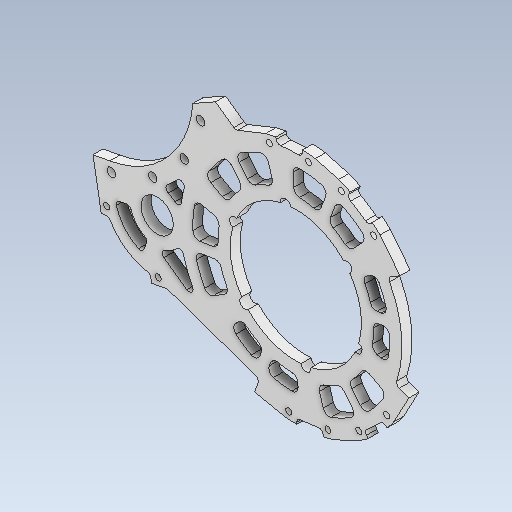
# Autodesk Inventor part: motor_h_2
Saved by Autodesk Inventor 2020 (Build 240168000, 168)
## iProperties
Created: 2020-07-14
Part Number: motor_h_2
Material: ABS Plastic
Document SubType Name: Modeling
Designer: psrobotics
Density: 1.06 g/cm^3
Appearance: Smooth - White
Author: psrobotics
Autodesk Inventor part; units mm, degrees
(part 1 of 2)
ref_plane "YZ Plane" through (0, 0, 0) normal (1, 0, 0) x (0, 1, 0)
ref_plane "XZ Plane" through (0, 0, 0) normal (0, 1, 0) x (-1, 0, 0)
ref_plane "XY Plane" through (0, 0, 0) normal (0, 0, 1) x (1, 0, 0)
sketch "Sketch1" plane through (0, 0, 0) normal (0, 0, 1) x (1, 0, 0)
  circle A0 centre (12.2297, 10.2049) radius 2.05 projected
  circle A1 centre (28.1949, -0.8291) radius 2.05 projected
  circle A2 centre (-4.0964, 14.5795) radius 2.05 projected
  circle A3 centre (-23.4396, 13.0063) radius 2.05 projected
  line L0 (35.1261, -15.125) -> (41.2511, -11.5887) projected
  line L1 (31.3473, 0.9908) -> (41.2511, -11.5887) projected
  arc A4 (31.3473, 0.9908) -> (27.4962, 4.4629) centre (-10.3402, -41.375) ccw projected
  line L2 (26.8782, 3.7142) -> (27.4962, 4.4629) projected
  arc A5 (24.1161, 3.4024) -> (26.8782, 3.7142) centre (25.3358, 4.9874) ccw projected
  arc A6 (24.1161, 3.4024) -> (16.8075, 8.1755) centre (-10.3402, -41.375) ccw projected
  arc A7 (15.9827, 10.8299) -> (16.8075, 8.1755) centre (17.7685, 9.9295) ccw projected
  line L3 (16.5842, 12.0228) -> (15.9827, 10.8299) projected
  arc A8 (16.5842, 12.0228) -> (10.8551, 14.5447) centre (-10.3402, -41.375) ccw projected
  line L4 (10.8551, 14.5447) -> (-0.736, 17.6505) projected
  arc A9 (-0.736, 17.6505) -> (-6.9585, 18.3311) centre (-10.3402, -41.375) ccw projected
  line L5 (-6.9585, 18.3311) -> (-7.034, 16.9972) projected
  arc A10 (-9.0756, 15.1108) -> (-7.034, 16.9972) centre (-9.0308, 17.1103) ccw projected
  arc A11 (-9.0756, 15.1108) -> (-17.7916, 14.6315) centre (-10.3402, -41.375) ccw projected
  arc A12 (-20.0277, 16.2826) -> (-17.7916, 14.6315) centre (-18.0553, 16.614) ccw projected
  line L6 (-20.0277, 16.2826) -> (-20.1886, 17.24) projected
  arc A13 (-20.1886, 17.24) -> (-25.2597, 16.1586) centre (-10.3402, -41.375) ccw projected
  line L7 (-25.2597, 16.1586) -> (-40.1265, 10.2163) projected
  line L8 (-40.1265, 10.2163) -> (-36.5902, 4.0913) projected
  arc A14 (35.1261, -15.125) -> (-36.5902, 4.0913) centre (-10.3402, -41.375) ccw projected
  circle A15 centre (5.5251, -95.3952) radius 2.05 projected
  circle A16 centre (-13.7974, -97.2048) radius 2.05 projected
  circle A17 centre (20.8436, -88.2521) radius 2.05 projected
  circle A18 centre (34.6501, -74.6133) radius 2.05 projected
  line L9 (-28.2963, -90.7089) -> (-30.7152, -97.3549) projected
  line L10 (-15.0425, -100.6253) -> (-30.7152, -97.3549) projected
  arc A19 (-15.0425, -100.6253) -> (-9.8606, -100.8097) centre (-10.3402, -41.375) ccw projected
  line L11 (-9.8684, -99.8389) -> (-9.8606, -100.8097) projected
  arc A20 (-7.953, -97.8245) -> (-9.8684, -99.8389) centre (-7.8685, -99.8228) ccw projected
  arc A21 (-7.953, -97.8245) -> (0.7138, -96.7831) centre (-10.3402, -41.375) ccw projected
  arc A22 (3.052, -98.2863) -> (0.7138, -96.7831) centre (1.1051, -98.7445) ccw projected
  line L12 (3.358, -99.5868) -> (3.052, -98.2863) projected
  arc A23 (3.358, -99.5868) -> (9.3677, -97.836) centre (-10.3402, -41.375) ccw projected
  line L13 (9.3677, -97.836) -> (20.2434, -92.7646) projected
  arc A24 (20.2434, -92.7646) -> (25.4476, -89.2862) centre (-10.3402, -41.375) ccw projected
  line L14 (25.4476, -89.2862) -> (24.6481, -88.2159) projected
  arc A25 (24.9994, -85.4585) -> (24.6481, -88.2159) centre (26.2504, -87.019) ccw projected
  arc A26 (24.9994, -85.4585) -> (31.3681, -79.4888) centre (-10.3402, -41.375) ccw projected
  arc A27 (34.1424, -79.3163) -> (31.3681, -79.4888) centre (32.8445, -80.838) ccw projected
  line L15 (34.1424, -79.3163) -> (34.8811, -79.9463) projected
  arc A28 (34.8811, -79.9463) -> (38.0707, -75.8583) centre (-10.3402, -41.375) ccw projected
  line L16 (38.0707, -75.8583) -> (45.6397, -61.75) projected
  line L17 (45.6397, -61.75) -> (38.9936, -59.3311) projected
  arc A29 (-28.2963, -90.7089) -> (38.9936, -59.3311) centre (-10.3402, -41.375) ccw projected
  circle A30 centre (-103.9086, -54.247) radius 2.1 projected
  circle A31 centre (-78.4226, -72.0925) radius 2.1 projected
  line L18 (-101.1564, -49.7) -> (-108.0501, -50.9156) projected
  line L19 (-107.6019, -53.4573) -> (-108.0501, -50.9156) projected
  line L20 (-106.6609, -58.794) -> (-107.6019, -53.4573) projected
  line L21 (-103.0049, -58.1494) -> (-106.6609, -58.794) projected
  arc A32 (-103.0049, -58.1494) -> (-96.5394, -66.3187) centre (-78.9982, -45.7929) ccw projected
  arc A33 (-96.5394, -66.3187) -> (-92.2867, -69.2965) centre (-78.9982, -45.7929) ccw projected
  arc A34 (-92.2867, -69.2965) -> (-82.3987, -72.578) centre (-78.9982, -45.7929) ccw projected
  line L22 (-82.3987, -72.578) -> (-81.7541, -76.234) projected
  line L23 (-81.7541, -76.234) -> (-76.4173, -75.2929) projected
  line L24 (-76.4173, -75.2929) -> (-73.8756, -74.8448) projected
  line L25 (-73.8756, -74.8448) -> (-75.0911, -67.9511) projected
  arc A35 (-101.1564, -49.7) -> (-75.0911, -67.9511) centre (-78.9982, -45.7929) ccw projected
  circle A36 centre (-111.1209, 15.0476) radius 45.5 projected
  arc A37 (-77.155, 49.6681) -> (-159.3589, 20.0812) centre (-111.1209, 15.0476) ccw projected
  circle A38 centre (-111.1209, 15.0476) radius 50
  circle A39 centre (-78.9982, -45.7929) radius 22.5
  circle A40 centre (-10.3402, -41.375) radius 52.5
  line L26 (-108.0501, -50.9156) -> (-110.8649, -34.9517)
  line L27 (-28.2963, -90.7089) -> (-73.8756, -74.8448)
  line L28 (-40.1265, 10.2163) -> (-62.337, 26.0083)
  line L29 (-88.8382, 29.4985) -> (-25.0902, -15.8273) projected
  point P0 (0, 0)
  dimension "d0" = 100
  dimension "d1" = 45
  dimension "d2" = 105
  constraints: 6 end point, 3 centre point, 3 coincident, 2 point on circle, 1 collinear, 1 parallel
  measures "d0" diameter of A38
  measures "d1" diameter of A39
  measures "d2" diameter of A40
extrude "Extrusion1" add sketch "Sketch1" along normal blind 5 contours A0 | A1 | A2 | A3 | A14 L8 L7 A13 L6 A12 A11 A10 L5 A9 L4 A8 L3 A7 A6 A5 L2 A4 L1 L0 | A40 A29 A39 A14 | A40 L29 A38 L28 L8 | A40 A39 A38 L29 | L17 L16 A28 L15 A27 A26 A25 L14 A24 L13 A23 L12 A22 A21 A20 L11 A19 L10 L9 A29 | A40 A39 A35 A38 | A39 A40 | L27 L25 A39 A40 | A38 A39 L18 L26 | L24 L23 L22 A34 A33 A32 L21 L20 L19 L18 A35 L25 | A15 | A16 | A17 | A18 | A30 | A31
sketch "Sketch2" plane through (0, 0, 5) normal (0, 0, 1) x (1, 0, 0)
  arc A0 (-20.0277, 16.2826) -> (-17.7916, 14.6315) centre (-18.0553, 16.614) ccw projected
  line L0 (-20.0277, 16.2826) -> (-20.1886, 17.24) projected
  arc A1 (-20.1886, 17.24) -> (-25.2597, 16.1586) centre (-10.3402, -41.375) ccw projected
  line L1 (-25.2597, 16.1586) -> (-40.1265, 10.2163) projected
  line L2 (-40.1265, 10.2163) -> (-62.337, 26.0083) projected
  arc A2 (-110.8649, -34.9517) -> (-62.337, 26.0083) centre (-111.1209, 15.0476) ccw projected
  line L3 (-110.8649, -34.9517) -> (-106.6609, -58.794) projected
  line L4 (-106.6609, -58.794) -> (-103.0049, -58.1494) projected
  arc A3 (-103.0049, -58.1494) -> (-82.3987, -72.578) centre (-78.9982, -45.7929) ccw projected
  line L5 (-82.3987, -72.578) -> (-81.7541, -76.234) projected
  line L6 (-81.7541, -76.234) -> (-73.8756, -74.8448) projected
  line L7 (-73.8756, -74.8448) -> (-28.2963, -90.7089) projected
  line L8 (-28.2963, -90.7089) -> (-30.7152, -97.3549) projected
  line L9 (-30.7152, -97.3549) -> (-15.0425, -100.6253) projected
  arc A4 (-15.0425, -100.6253) -> (-9.8606, -100.8097) centre (-10.3402, -41.375) ccw projected
  line L10 (-9.8606, -100.8097) -> (-9.8684, -99.8389) projected
  arc A5 (-7.953, -97.8245) -> (-9.8684, -99.8389) centre (-7.8685, -99.8228) ccw projected
  arc A6 (-7.953, -97.8245) -> (0.7138, -96.7831) centre (-10.3402, -41.375) ccw projected
  arc A7 (3.052, -98.2863) -> (0.7138, -96.7831) centre (1.1051, -98.7445) ccw projected
  line L11 (3.052, -98.2863) -> (3.358, -99.5868) projected
  arc A8 (3.358, -99.5868) -> (9.3677, -97.836) centre (-10.3402, -41.375) ccw projected
  line L12 (9.3677, -97.836) -> (20.2434, -92.7646) projected
  arc A9 (20.2434, -92.7646) -> (25.4476, -89.2862) centre (-10.3402, -41.375) ccw projected
  line L13 (25.4476, -89.2862) -> (24.6481, -88.2159) projected
  arc A10 (24.9994, -85.4585) -> (24.6481, -88.2159) centre (26.2504, -87.019) ccw projected
  arc A11 (24.9994, -85.4585) -> (31.3681, -79.4888) centre (-10.3402, -41.375) ccw projected
  arc A12 (34.1424, -79.3163) -> (31.3681, -79.4888) centre (32.8445, -80.838) ccw projected
  line L14 (34.1424, -79.3163) -> (34.8811, -79.9463) projected
  arc A13 (34.8811, -79.9463) -> (38.0707, -75.8583) centre (-10.3402, -41.375) ccw projected
  line L15 (38.0707, -75.8583) -> (45.6397, -61.75) projected
  line L16 (45.6397, -61.75) -> (38.9936, -59.3311) projected
  arc A14 (38.9936, -59.3311) -> (35.1261, -15.125) centre (-10.3402, -41.375) ccw projected
  line L17 (35.1261, -15.125) -> (41.2511, -11.5887) projected
  line L18 (41.2511, -11.5887) -> (31.3473, 0.9908) projected
  arc A15 (31.3473, 0.9908) -> (27.4962, 4.4629) centre (-10.3402, -41.375) ccw projected
  line L19 (27.4962, 4.4629) -> (26.8782, 3.7142) projected
  arc A16 (24.1161, 3.4024) -> (26.8782, 3.7142) centre (25.3358, 4.9874) ccw projected
  arc A17 (24.1161, 3.4024) -> (16.8075, 8.1755) centre (-10.3402, -41.375) ccw projected
  arc A18 (15.9827, 10.8299) -> (16.8075, 8.1755) centre (17.7685, 9.9295) ccw projected
  line L20 (15.9827, 10.8299) -> (16.5842, 12.0228) projected
  arc A19 (16.5842, 12.0228) -> (10.8551, 14.5447) centre (-10.3402, -41.375) ccw projected
  line L21 (10.8551, 14.5447) -> (-0.736, 17.6505) projected
  arc A20 (-0.736, 17.6505) -> (-6.9585, 18.3311) centre (-10.3402, -41.375) ccw projected
  line L22 (-6.9585, 18.3311) -> (-7.034, 16.9972) projected
  arc A21 (-9.0756, 15.1108) -> (-7.034, 16.9972) centre (-9.0308, 17.1103) ccw projected
  arc A22 (-9.0756, 15.1108) -> (-17.7916, 14.6315) centre (-10.3402, -41.375) ccw projected
  line L23 (-111.1209, 15.0476) -> (-102.4384, -34.1927)
  line L24 (-102.4384, -34.1927) -> (-110.7406, -35.6566)
  line L25 (-110.8649, -34.9517) -> (-106.6609, -58.794) projected
  point P0 (0, 0)
  constraints: 4 end point, 2 perpendicular, 1 point on circle, 1 point on line
extrude "Extrusion2" cut sketch "Sketch2" against normal blind 5 contours L24 L3 A2
sketch "Sketch3" plane through (0, 0, 5) normal (0, 0, 1) x (1, 0, 0)
  circle A0 centre (-23.4396, 13.0063) radius 2.05 projected
  circle A1 centre (-4.0964, 14.5795) radius 2.05 projected
  circle A2 centre (12.2297, 10.2049) radius 2.05 projected
  circle A3 centre (28.1949, -0.8291) radius 2.05 projected
  circle A4 centre (34.6501, -74.6133) radius 2.05 projected
  circle A5 centre (20.8436, -88.2521) radius 2.05 projected
  circle A6 centre (5.5251, -95.3952) radius 2.05 projected
  circle A7 centre (-13.7974, -97.2048) radius 2.05 projected
  circle A8 centre (-78.4226, -72.0925) radius 2.1 projected
  circle A9 centre (-103.9086, -54.247) radius 2.1 projected
  point P0 (0, 0)
hole "Hole1" at (-23.4396, 13.0063, 5) at (-4.0964, 14.5795, 5) at (12.2297, 10.2049, 5) at (28.1949, -0.8291, 5) at (34.6501, -74.6133, 5) at (20.8436, -88.2521, 5) at (5.5251, -95.3952, 5) at (-13.7974, -97.2048, 5) at (-78.4226, -72.0925, 5) at (-103.9086, -54.247, 5) direction (0, 0, -1) diameter 3 depth 17
sketch "Sketch6" plane through (0, 0, 5) normal (0, 0, 1) x (1, 0, 0)
  circle A0 centre (-10.3402, -41.375) radius 4.075 projected
  circle A1 centre (-10.3402, -41.375) radius 32.5 projected
  circle A2 centre (-10.3402, -41.375) radius 32.5
  point P0 (0, 0)
  dimension "d16" = 65
  constraints: 1 centre point, 1 coincident
  measures "d16" diameter of A2
extrude "Extrusion4" cut sketch "Sketch6" against normal blind 5 contours A0 | A1
chamfer "Chamfer1" distance 15 angle 45 1 edges at (-62.337, 26.0083, 2.5)
sketch "Sketch7" plane through (0, 0, 5) normal (0, 0, 1) x (1, 0, 0)
  circle A0 centre (-78.9982, -45.7929) radius 4.075 projected
  circle A1 centre (-78.9982, -45.7929) radius 8
  point P0 (0, 0)
  dimension "d22" = 16
  constraints: 1 centre point, 1 coincident
  measures "d22" diameter of A1
extrude "Extrusion5" cut sketch "Sketch7" against normal blind 5 contours A0 | A1
sketch "Sketch8" plane through (0, 0, 5) normal (0, 0, 1) x (1, 0, 0)
  circle A0 centre (-78.9982, -45.7929) radius 8 projected
  line L0 (-61.2813, 11.0455) -> (-50.1121, 17.3163) projected
  arc A1 (-102.4384, -34.1927) -> (-61.2813, 11.0455) centre (-111.1209, 15.0476) ccw projected
  line L1 (-102.4384, -34.1927) -> (-110.7406, -35.6566) projected
  line L2 (-110.7406, -35.6566) -> (-106.6609, -58.794) projected
  line L3 (-106.6609, -58.794) -> (-103.0049, -58.1494) projected
  arc A2 (-103.0049, -58.1494) -> (-82.3987, -72.578) centre (-78.9982, -45.7929) ccw projected
  line L4 (-82.3987, -72.578) -> (-81.7541, -76.234) projected
  line L5 (-81.7541, -76.234) -> (-73.8756, -74.8448) projected
  line L6 (-73.8756, -74.8448) -> (-28.2963, -90.7089) projected
  line L7 (-28.2963, -90.7089) -> (-30.7152, -97.3549) projected
  line L8 (-30.7152, -97.3549) -> (-15.0425, -100.6253) projected
  arc A3 (-15.0425, -100.6253) -> (-9.8606, -100.8097) centre (-10.3402, -41.375) ccw projected
  line L9 (-9.8606, -100.8097) -> (-9.8684, -99.8389) projected
  arc A4 (-7.953, -97.8245) -> (-9.8684, -99.8389) centre (-7.8685, -99.8228) ccw projected
  arc A5 (-7.953, -97.8245) -> (0.7138, -96.7831) centre (-10.3402, -41.375) ccw projected
  arc A6 (3.052, -98.2863) -> (0.7138, -96.7831) centre (1.1051, -98.7445) ccw projected
  line L10 (3.052, -98.2863) -> (3.358, -99.5868) projected
  arc A7 (3.358, -99.5868) -> (9.3677, -97.836) centre (-10.3402, -41.375) ccw projected
  line L11 (9.3677, -97.836) -> (20.2434, -92.7646) projected
  arc A8 (20.2434, -92.7646) -> (25.4476, -89.2862) centre (-10.3402, -41.375) ccw projected
  line L12 (25.4476, -89.2862) -> (24.6481, -88.2159) projected
  arc A9 (24.9994, -85.4585) -> (24.6481, -88.2159) centre (26.2504, -87.019) ccw projected
  arc A10 (24.9994, -85.4585) -> (31.3681, -79.4888) centre (-10.3402, -41.375) ccw projected
  arc A11 (34.1424, -79.3163) -> (31.3681, -79.4888) centre (32.8445, -80.838) ccw projected
  line L13 (34.1424, -79.3163) -> (34.8811, -79.9463) projected
  arc A12 (34.8811, -79.9463) -> (38.0707, -75.8583) centre (-10.3402, -41.375) ccw projected
  line L14 (38.0707, -75.8583) -> (45.6397, -61.75) projected
  line L15 (45.6397, -61.75) -> (38.9936, -59.3311) projected
  arc A13 (38.9936, -59.3311) -> (35.1261, -15.125) centre (-10.3402, -41.375) ccw projected
  line L16 (35.1261, -15.125) -> (41.2511, -11.5887) projected
  line L17 (41.2511, -11.5887) -> (31.3473, 0.9908) projected
  arc A14 (31.3473, 0.9908) -> (27.4962, 4.4629) centre (-10.3402, -41.375) ccw projected
  line L18 (27.4962, 4.4629) -> (26.8782, 3.7142) projected
  arc A15 (24.1161, 3.4024) -> (26.8782, 3.7142) centre (25.3358, 4.9874) ccw projected
  arc A16 (24.1161, 3.4024) -> (16.8075, 8.1755) centre (-10.3402, -41.375) ccw projected
  arc A17 (15.9827, 10.8299) -> (16.8075, 8.1755) centre (17.7685, 9.9295) ccw projected
  line L19 (15.9827, 10.8299) -> (16.5842, 12.0228) projected
  arc A18 (16.5842, 12.0228) -> (10.8551, 14.5447) centre (-10.3402, -41.375) ccw projected
  line L20 (10.8551, 14.5447) -> (-0.736, 17.6505) projected
  arc A19 (-0.736, 17.6505) -> (-6.9585, 18.3311) centre (-10.3402, -41.375) ccw projected
  line L21 (-6.9585, 18.3311) -> (-7.034, 16.9972) projected
  arc A20 (-9.0756, 15.1108) -> (-7.034, 16.9972) centre (-9.0308, 17.1103) ccw projected
  arc A21 (-9.0756, 15.1108) -> (-17.7916, 14.6315) centre (-10.3402, -41.375) ccw projected
  arc A22 (-20.0277, 16.2826) -> (-17.7916, 14.6315) centre (-18.0553, 16.614) ccw projected
  line L22 (-20.0277, 16.2826) -> (-20.1886, 17.24) projected
  arc A23 (-20.1886, 17.24) -> (-25.2597, 16.1586) centre (-10.3402, -41.375) ccw projected
  line L23 (-25.2597, 16.1586) -> (-40.1265, 10.2163) projected
  line L24 (-40.1265, 10.2163) -> (-50.1121, 17.3163) projected
  circle A24 centre (-103.9086, -54.247) radius 1.5 projected
  circle A25 centre (-13.7974, -97.2048) radius 1.5 projected
  circle A26 centre (20.8436, -88.2521) radius 1.5 projected
  circle A27 centre (28.1949, -0.8291) radius 1.5 projected
  circle A28 centre (-4.0964, 14.5795) radius 1.5 projected
  circle A29 centre (-23.4396, 13.0063) radius 1.5 projected
  circle A30 centre (12.2297, 10.2049) radius 1.5 projected
  circle A31 centre (34.6501, -74.6133) radius 1.5 projected
  circle A32 centre (5.5251, -95.3952) radius 1.5 projected
  circle A33 centre (-78.4226, -72.0925) radius 1.5 projected
  circle A34 centre (-10.3402, -41.375) radius 32.5 projected
  circle A35 centre (-111.1209, 15.0476) radius 50
  circle A36 centre (-111.1209, 15.0476) radius 59
  line L25 (-110.7406, -35.6566) -> (-102.4384, -34.1927) projected
  line L26 (-111.1209, 15.0476) -> (-102.4384, -34.1927)
  line L27 (-102.4384, -34.1927) -> (-100.8756, -43.056)
  circle A37 centre (-101.657, -38.6244) radius 2.1
  circle A38 centre (-81.1726, -30.4864) radius 2.1
  circle A39 centre (-65.5868, -14.9006) radius 2.1
  circle A40 centre (-57.4488, 5.5838) radius 2.1
  point P0 (0, 0)
  dimension "d26" = 118
  dimension "d25" = 100
  dimension "d27" = 4.2
  dimension "d30" = 70
  constraints: 5 centre point, 4 end point, 2 coincident, 1 midpoint, 1 perpendicular, 1 point on line, 10 other
  measures "d25" diameter of A35
  measures "d27" diameter of A37
extrude "Extrusion6" cut sketch "Sketch8" against normal blind 5 contours A37 L27 | L27 A37 | A38 | A39 | A40
sketch "Sketch10" plane through (0, 0, 5) normal (0, 0, 1) x (1, 0, 0)
  circle A0 centre (-10.3402, -41.375) radius 32.5 projected
  circle A1 centre (-81.1726, -30.4864) radius 2.1 projected
  circle A2 centre (-65.5868, -14.9006) radius 2.1 projected
  circle A3 centre (-101.657, -38.6244) radius 2.1 projected
  circle A4 centre (-57.4488, 5.5838) radius 2.1 projected
  circle A5 centre (-78.9982, -45.7929) radius 8 projected
  line L0 (-61.2813, 11.0455) -> (-50.1121, 17.3163) projected
  arc A6 (-102.4384, -34.1927) -> (-61.2813, 11.0455) centre (-111.1209, 15.0476) ccw projected
  line L1 (-102.4384, -34.1927) -> (-110.7406, -35.6566) projected
  line L2 (-110.7406, -35.6566) -> (-106.6609, -58.794) projected
  line L3 (-106.6609, -58.794) -> (-103.0049, -58.1494) projected
  arc A7 (-103.0049, -58.1494) -> (-82.3987, -72.578) centre (-78.9982, -45.7929) ccw projected
  line L4 (-82.3987, -72.578) -> (-81.7541, -76.234) projected
  line L5 (-81.7541, -76.234) -> (-73.8756, -74.8448) projected
  line L6 (-73.8756, -74.8448) -> (-28.2963, -90.7089) projected
  line L7 (-28.2963, -90.7089) -> (-30.7152, -97.3549) projected
  line L8 (-30.7152, -97.3549) -> (-15.0425, -100.6253) projected
  arc A8 (-15.0425, -100.6253) -> (-9.8606, -100.8097) centre (-10.3402, -41.375) ccw projected
  line L9 (-9.8606, -100.8097) -> (-9.8684, -99.8389) projected
  arc A9 (-7.953, -97.8245) -> (-9.8684, -99.8389) centre (-7.8685, -99.8228) ccw projected
  arc A10 (-7.953, -97.8245) -> (0.7138, -96.7831) centre (-10.3402, -41.375) ccw projected
  arc A11 (3.052, -98.2863) -> (0.7138, -96.7831) centre (1.1051, -98.7445) ccw projected
  line L10 (3.052, -98.2863) -> (3.358, -99.5868) projected
  arc A12 (3.358, -99.5868) -> (9.3677, -97.836) centre (-10.3402, -41.375) ccw projected
  line L11 (9.3677, -97.836) -> (20.2434, -92.7646) projected
  arc A13 (20.2434, -92.7646) -> (25.4476, -89.2862) centre (-10.3402, -41.375) ccw projected
  line L12 (25.4476, -89.2862) -> (24.6481, -88.2159) projected
  arc A14 (24.9994, -85.4585) -> (24.6481, -88.2159) centre (26.2504, -87.019) ccw projected
  arc A15 (24.9994, -85.4585) -> (31.3681, -79.4888) centre (-10.3402, -41.375) ccw projected
  arc A16 (34.1424, -79.3163) -> (31.3681, -79.4888) centre (32.8445, -80.838) ccw projected
  line L13 (34.1424, -79.3163) -> (34.8811, -79.9463) projected
  arc A17 (34.8811, -79.9463) -> (38.0707, -75.8583) centre (-10.3402, -41.375) ccw projected
  line L14 (38.0707, -75.8583) -> (45.6397, -61.75) projected
  line L15 (45.6397, -61.75) -> (38.9936, -59.3311) projected
  arc A18 (38.9936, -59.3311) -> (35.1261, -15.125) centre (-10.3402, -41.375) ccw projected
  line L16 (35.1261, -15.125) -> (41.2511, -11.5887) projected
  line L17 (41.2511, -11.5887) -> (31.3473, 0.9908) projected
  arc A19 (31.3473, 0.9908) -> (27.4962, 4.4629) centre (-10.3402, -41.375) ccw projected
  line L18 (27.4962, 4.4629) -> (26.8782, 3.7142) projected
  arc A20 (24.1161, 3.4024) -> (26.8782, 3.7142) centre (25.3358, 4.9874) ccw projected
  arc A21 (24.1161, 3.4024) -> (16.8075, 8.1755) centre (-10.3402, -41.375) ccw projected
  arc A22 (15.9827, 10.8299) -> (16.8075, 8.1755) centre (17.7685, 9.9295) ccw projected
  line L19 (15.9827, 10.8299) -> (16.5842, 12.0228) projected
  arc A23 (16.5842, 12.0228) -> (10.8551, 14.5447) centre (-10.3402, -41.375) ccw projected
  line L20 (10.8551, 14.5447) -> (-0.736, 17.6505) projected
  arc A24 (-0.736, 17.6505) -> (-6.9585, 18.3311) centre (-10.3402, -41.375) ccw projected
  line L21 (-6.9585, 18.3311) -> (-7.034, 16.9972) projected
  arc A25 (-9.0756, 15.1108) -> (-7.034, 16.9972) centre (-9.0308, 17.1103) ccw projected
  arc A26 (-9.0756, 15.1108) -> (-17.7916, 14.6315) centre (-10.3402, -41.375) ccw projected
  arc A27 (-20.0277, 16.2826) -> (-17.7916, 14.6315) centre (-18.0553, 16.614) ccw projected
  line L22 (-20.0277, 16.2826) -> (-20.1886, 17.24) projected
  arc A28 (-20.1886, 17.24) -> (-25.2597, 16.1586) centre (-10.3402, -41.375) ccw projected
  line L23 (-25.2597, 16.1586) -> (-40.1265, 10.2163) projected
  line L24 (-40.1265, 10.2163) -> (-50.1121, 17.3163) projected
  circle A29 centre (-103.9086, -54.247) radius 1.5 projected
  circle A30 centre (-13.7974, -97.2048) radius 1.5 projected
  circle A31 centre (20.8436, -88.2521) radius 1.5 projected
  circle A32 centre (28.1949, -0.8291) radius 1.5 projected
  circle A33 centre (-4.0964, 14.5795) radius 1.5 projected
  circle A34 centre (-23.4396, 13.0063) radius 1.5 projected
  circle A35 centre (12.2297, 10.2049) radius 1.5 projected
  circle A36 centre (34.6501, -74.6133) radius 1.5 projected
  circle A37 centre (5.5251, -95.3952) radius 1.5 projected
  circle A38 centre (-78.4226, -72.0925) radius 1.5 projected
  circle A39 centre (-10.3402, -41.375) radius 32.5 projected
  circle A40 centre (28.1949, -0.8291) radius 1.5 projected
  line L25 (-10.3402, -41.375) -> (28.1949, -0.8291)
  circle A41 centre (-10.3402, -41.375) radius 32.5
  circle A42 centre (-10.3402, -41.375) radius 38.5
  circle A43 centre (-10.3402, -41.375) radius 46.5
  circle A44 centre (-10.3402, -41.375) radius 51
  line L26 (-10.3402, -41.375) -> (39.2416, -53.3183)
  line L27 (-10.3402, -41.375) -> (33.1646, -14.7606)
  line L28 (-10.3402, -41.375) -> (-11.6366, 9.6085)
  line L29 (-10.3402, -41.375) -> (24.7939, -4.4075)
  line L30 (-10.3402, -41.375) -> (-55.1414, -17.0059)
  line L31 (-10.3402, -41.375) -> (-24.7879, 7.5358)
  line L32 (-10.3402, -41.375) -> (-53.8451, -67.9894)
  line L33 (-10.3402, -41.375) -> (-59.922, -29.4317)
  line L34 (-10.3402, -41.375) -> (-9.0439, -92.3585)
  line L35 (-10.3402, -41.375) -> (-45.4743, -78.3425)
  line L36 (-10.3402, -41.375) -> (34.461, -65.7441)
  line L37 (-10.3402, -41.375) -> (4.1075, -90.2858)
  point P0 (0, 0)
  point P1 (-11.3188, -2.8874)
  point P2 (16.1826, -13.4682)
  point P3 (24.7939, -4.4075)
  point P4 (-44.1607, -22.9787)
  point P5 (-21.2468, -4.4522)
  point P6 (-43.1821, -61.4663)
  point P7 (-47.7696, -32.359)
  point P8 (-36.863, -69.2818)
  point P9 (-42.3743, -75.0806)
  point P10 (-9.1582, -87.86)
  point P11 (-9.3616, -79.8626)
  point P12 (23.4803, -59.7713)
  point P13 (0.5664, -78.2978)
  point P14 (29.326, -17.1089)
  point P15 (22.5017, -21.2837)
  point P16 (27.0892, -50.391)
  point P17 (34.8667, -52.2645)
  dimension "d38" = 65
  dimension "d39" = 77
  dimension "d40" = 93
  dimension "d41" = 102
  dimension "d42" = 60
  dimension "d43" = 15
  dimension "d46" = 360
  constraints: 26 end point, 4 centre point, 4 coincident, 2 point on circle, 31 other
  measures "d38" diameter of A41
  measures "d39" diameter of A42
  measures "d40" diameter of A43
  measures "d41" diameter of A44
  measures "d42" angle of L25 L26
  measures "d43" angle of L25 L27
extrude "Extrusion8" cut sketch "Sketch10" against normal blind 5 contours L27 A43 L26 A42 | A42 L28 A43 L25 | L36 A43 L37 A42 | A43 L28 A44 L25 | L30 A43 L31 A42 | L32 A43 L33 A42 | L34 A43 L35 A42 | L36 A44 L37 A43 | L30 A44 L31 A43 | L32 A44 L33 A43
sketch "Sketch11" plane through (0, 0, 5) normal (0, 0, 1) x (1, 0, 0)
  line L0 (-9.3616, -79.8626) -> (-9.1582, -87.86) projected
  arc A0 (-42.3743, -75.0806) -> (-9.1582, -87.86) centre (-10.3402, -41.375) ccw projected
  line L1 (-42.3743, -75.0806) -> (-36.863, -69.2818) projected
  arc A1 (-36.863, -69.2818) -> (-9.3616, -79.8626) centre (-10.3402, -41.375) ccw projected
  arc A2 (24.7939, -4.4075) -> (-11.6366, 9.6085) centre (-10.3402, -41.375) ccw projected
  line L2 (24.7939, -4.4075) -> (16.1826, -13.4682) projected
  arc A3 (16.1826, -13.4682) -> (-11.3188, -2.8874) centre (-10.3402, -41.375) ccw projected
  line L3 (-11.3188, -2.8874) -> (-11.6366, 9.6085) projected
  line L4 (23.4803, -59.7713) -> (34.461, -65.7441) projected
  arc A4 (4.1075, -90.2858) -> (34.461, -65.7441) centre (-10.3402, -41.375) ccw projected
  line L5 (4.1075, -90.2858) -> (0.5664, -78.2978) projected
  arc A5 (0.5664, -78.2978) -> (23.4803, -59.7713) centre (-10.3402, -41.375) ccw projected
  arc A6 (-47.7696, -32.359) -> (-43.1821, -61.4663) centre (-10.3402, -41.375) ccw projected
  line L6 (-43.1821, -61.4663) -> (-53.8451, -67.9894) projected
  arc A7 (-59.922, -29.4317) -> (-53.8451, -67.9894) centre (-10.3402, -41.375) ccw projected
  line L7 (-59.922, -29.4317) -> (-47.7696, -32.359) projected
  arc A8 (-21.2468, -4.4522) -> (-44.1607, -22.9787) centre (-10.3402, -41.375) ccw projected
  line L8 (-44.1607, -22.9787) -> (-55.1414, -17.0059) projected
  arc A9 (-24.7879, 7.5358) -> (-55.1414, -17.0059) centre (-10.3402, -41.375) ccw projected
  line L9 (-24.7879, 7.5358) -> (-21.2468, -4.4522) projected
  arc A10 (34.8667, -52.2645) -> (29.326, -17.1089) centre (-10.3402, -41.375) ccw projected
  line L10 (34.8667, -52.2645) -> (27.0892, -50.391) projected
  arc A11 (27.0892, -50.391) -> (22.5017, -21.2837) centre (-10.3402, -41.375) ccw projected
  line L11 (22.5017, -21.2837) -> (29.326, -17.1089) projected
  circle A12 centre (-81.1726, -30.4864) radius 2.1 projected
  circle A13 centre (-65.5868, -14.9006) radius 2.1 projected
  circle A14 centre (-101.657, -38.6244) radius 2.1 projected
  circle A15 centre (-57.4488, 5.5838) radius 2.1 projected
  circle A16 centre (-78.9982, -45.7929) radius 8 projected
  line L12 (-61.2813, 11.0455) -> (-50.1121, 17.3163) projected
  arc A17 (-102.4384, -34.1927) -> (-61.2813, 11.0455) centre (-111.1209, 15.0476) ccw projected
  line L13 (-102.4384, -34.1927) -> (-110.7406, -35.6566) projected
  line L14 (-110.7406, -35.6566) -> (-106.6609, -58.794) projected
  line L15 (-106.6609, -58.794) -> (-103.0049, -58.1494) projected
  arc A18 (-103.0049, -58.1494) -> (-82.3987, -72.578) centre (-78.9982, -45.7929) ccw projected
  line L16 (-82.3987, -72.578) -> (-81.7541, -76.234) projected
  line L17 (-81.7541, -76.234) -> (-73.8756, -74.8448) projected
  line L18 (-73.8756, -74.8448) -> (-28.2963, -90.7089) projected
  line L19 (-28.2963, -90.7089) -> (-30.7152, -97.3549) projected
  line L20 (-30.7152, -97.3549) -> (-15.0425, -100.6253) projected
  arc A19 (-15.0425, -100.6253) -> (-9.8606, -100.8097) centre (-10.3402, -41.375) ccw projected
  line L21 (-9.8606, -100.8097) -> (-9.8684, -99.8389) projected
  arc A20 (-7.953, -97.8245) -> (-9.8684, -99.8389) centre (-7.8685, -99.8228) ccw projected
  arc A21 (-7.953, -97.8245) -> (0.7138, -96.7831) centre (-10.3402, -41.375) ccw projected
  arc A22 (3.052, -98.2863) -> (0.7138, -96.7831) centre (1.1051, -98.7445) ccw projected
  line L22 (3.052, -98.2863) -> (3.358, -99.5868) projected
  arc A23 (3.358, -99.5868) -> (9.3677, -97.836) centre (-10.3402, -41.375) ccw projected
  line L23 (9.3677, -97.836) -> (20.2434, -92.7646) projected
  arc A24 (20.2434, -92.7646) -> (25.4476, -89.2862) centre (-10.3402, -41.375) ccw projected
  line L24 (25.4476, -89.2862) -> (24.6481, -88.2159) projected
  arc A25 (24.9994, -85.4585) -> (24.6481, -88.2159) centre (26.2504, -87.019) ccw projected
  arc A26 (24.9994, -85.4585) -> (31.3681, -79.4888) centre (-10.3402, -41.375) ccw projected
  arc A27 (34.1424, -79.3163) -> (31.3681, -79.4888) centre (32.8445, -80.838) ccw projected
  line L25 (34.1424, -79.3163) -> (34.8811, -79.9463) projected
  arc A28 (34.8811, -79.9463) -> (38.0707, -75.8583) centre (-10.3402, -41.375) ccw projected
  line L26 (38.0707, -75.8583) -> (45.6397, -61.75) projected
  line L27 (45.6397, -61.75) -> (38.9936, -59.3311) projected
  arc A29 (38.9936, -59.3311) -> (35.1261, -15.125) centre (-10.3402, -41.375) ccw projected
  line L28 (35.1261, -15.125) -> (41.2511, -11.5887) projected
  line L29 (41.2511, -11.5887) -> (31.3473, 0.9908) projected
  arc A30 (31.3473, 0.9908) -> (27.4962, 4.4629) centre (-10.3402, -41.375) ccw projected
  line L30 (27.4962, 4.4629) -> (26.8782, 3.7142) projected
  arc A31 (24.1161, 3.4024) -> (26.8782, 3.7142) centre (25.3358, 4.9874) ccw projected
  arc A32 (24.1161, 3.4024) -> (16.8075, 8.1755) centre (-10.3402, -41.375) ccw projected
  arc A33 (15.9827, 10.8299) -> (16.8075, 8.1755) centre (17.7685, 9.9295) ccw projected
  line L31 (15.9827, 10.8299) -> (16.5842, 12.0228) projected
  arc A34 (16.5842, 12.0228) -> (10.8551, 14.5447) centre (-10.3402, -41.375) ccw projected
  line L32 (10.8551, 14.5447) -> (-0.736, 17.6505) projected
  arc A35 (-0.736, 17.6505) -> (-6.9585, 18.3311) centre (-10.3402, -41.375) ccw projected
  line L33 (-6.9585, 18.3311) -> (-7.034, 16.9972) projected
  arc A36 (-9.0756, 15.1108) -> (-7.034, 16.9972) centre (-9.0308, 17.1103) ccw projected
  arc A37 (-9.0756, 15.1108) -> (-17.7916, 14.6315) centre (-10.3402, -41.375) ccw projected
  arc A38 (-20.0277, 16.2826) -> (-17.7916, 14.6315) centre (-18.0553, 16.614) ccw projected
  line L34 (-20.0277, 16.2826) -> (-20.1886, 17.24) projected
  arc A39 (-20.1886, 17.24) -> (-25.2597, 16.1586) centre (-10.3402, -41.375) ccw projected
  line L35 (-25.2597, 16.1586) -> (-40.1265, 10.2163) projected
  line L36 (-40.1265, 10.2163) -> (-50.1121, 17.3163) projected
  circle A40 centre (-103.9086, -54.247) radius 1.5 projected
  circle A41 centre (-13.7974, -97.2048) radius 1.5 projected
  circle A42 centre (20.8436, -88.2521) radius 1.5 projected
  circle A43 centre (28.1949, -0.8291) radius 1.5 projected
  circle A44 centre (-4.0964, 14.5795) radius 1.5 projected
  circle A45 centre (-23.4396, 13.0063) radius 1.5 projected
  circle A46 centre (12.2297, 10.2049) radius 1.5 projected
  circle A47 centre (34.6501, -74.6133) radius 1.5 projected
  circle A48 centre (5.5251, -95.3952) radius 1.5 projected
  circle A49 centre (-78.4226, -72.0925) radius 1.5 projected
  circle A50 centre (-10.3402, -41.375) radius 32.5 projected
  line L37 (-10.3402, -41.375) -> (27.6903, -35.3811)
  line L38 (27.6903, -35.3811) -> (35.5928, -34.1356)
  arc A51 (34.8667, -52.2645) -> (29.326, -17.1089) centre (-10.3402, -41.375) ccw projected
  line L39 (35.5928, -34.1356) -> (27.6903, -35.3811) construction
  line L40 (35.2036, -31.6661) -> (27.3011, -32.9116)
  line L41 (28.0796, -37.8506) -> (35.982, -36.6051)
  arc A52 (35.982, -36.6051) -> (35.2036, -31.6661) centre (35.5928, -34.1356) ccw
  arc A53 (27.3011, -32.9116) -> (28.0796, -37.8506) centre (27.6903, -35.3811) ccw
  arc A54 (0.5664, -78.2978) -> (23.4803, -59.7713) centre (-10.3402, -41.375) ccw projected
  line L42 (13.8659, -71.3135) -> (21.7251, -81.0338)
  arc A55 (4.1075, -90.2858) -> (34.461, -65.7441) centre (-10.3402, -41.375) ccw projected
  line L43 (13.8659, -71.3135) -> (21.7251, -81.0338) construction
  line L44 (11.9219, -72.8853) -> (19.781, -82.6056)
  line L45 (23.6691, -79.4619) -> (15.81, -69.7417)
  arc A56 (15.81, -69.7417) -> (11.9219, -72.8853) centre (13.8659, -71.3135) ccw
  arc A57 (19.781, -82.6056) -> (23.6691, -79.4619) centre (21.7251, -81.0338) ccw
  line L46 (3.4842, -5.4426) -> (7.9727, 6.2237) construction
  line L47 (5.8175, -6.3403) -> (10.3059, 5.326)
  line L48 (5.6394, 7.1214) -> (1.1509, -4.5449)
  arc A58 (1.1509, -4.5449) -> (5.8175, -6.3403) centre (3.4842, -5.4426) ccw
  arc A59 (10.3059, 5.326) -> (5.6394, 7.1214) centre (7.9727, 6.2237) ccw
  line L49 (-34.5464, -11.4365) -> (-42.4055, -1.7162) construction
  arc A60 (-24.7879, 7.5358) -> (-55.1414, -17.0059) centre (-10.3402, -41.375) ccw projected
  line L50 (-32.6023, -9.8647) -> (-40.4614, -0.1444)
  line L51 (-44.3495, -3.2881) -> (-36.4904, -13.0083)
  arc A61 (-36.4904, -13.0083) -> (-32.6023, -9.8647) centre (-34.5464, -11.4365) ccw
  arc A62 (-40.4614, -0.1444) -> (-44.3495, -3.2881) centre (-42.4055, -1.7162) ccw
  arc A63 (-47.7696, -32.359) -> (-43.1821, -61.4663) centre (-10.3402, -41.375) ccw projected
  line L52 (-48.3708, -47.3689) -> (-60.7184, -49.315) construction
  arc A64 (-59.922, -29.4317) -> (-53.8451, -67.9894) centre (-10.3402, -41.375) ccw projected
  line L53 (-48.76, -44.8994) -> (-61.1076, -46.8454)
  line L54 (-60.3291, -51.7845) -> (-47.9816, -49.8384)
  arc A65 (-47.9816, -49.8384) -> (-48.76, -44.8994) centre (-48.3708, -47.3689) ccw
  arc A66 (-61.1076, -46.8454) -> (-60.3291, -51.7845) centre (-60.7184, -49.315) ccw
  arc A67 (-36.863, -69.2818) -> (-9.3616, -79.8626) centre (-10.3402, -41.375) ccw projected
  line L55 (-24.1646, -77.3074) -> (-27.0372, -84.7738) construction
  line L56 (-26.4979, -76.4097) -> (-29.3705, -83.8761)
  line L57 (-24.704, -85.6715) -> (-21.8314, -78.2051)
  arc A68 (-21.8314, -78.2051) -> (-26.4979, -76.4097) centre (-24.1646, -77.3074) ccw
  arc A69 (-29.3705, -83.8761) -> (-24.704, -85.6715) centre (-27.0372, -84.7738) ccw
  point P0 (0, 0)
  point P1 (31.6416, -34.7584)
  point P2 (17.7955, -76.1736)
  point P3 (5.7284, 0.3905)
  point P4 (-38.4759, -6.5764)
  point P5 (-54.5446, -48.3419)
  point P6 (-25.6009, -81.0406)
  point P7 (5.7871, -6.4156)
  point P8 (10.2839, 5.2688)
  point P9 (5.6174, 7.0642)
  point P10 (1.123, -4.6212)
  point P11 (-32.5523, -9.9286)
  point P12 (-40.4229, -0.1921)
  point P13 (-44.311, -3.3357)
  point P14 (-36.4384, -13.0706)
  point P15 (-48.6796, -44.888)
  point P16 (-61.047, -46.8359)
  point P17 (-60.2686, -51.7749)
  point P18 (-47.9016, -49.8245)
  point P19 (-26.4675, -76.3344)
  point P20 (-29.3464, -83.8134)
  point P21 (-24.6798, -85.6088)
  point P22 (-21.8035, -78.1288)
  point P23 (15.7579, -69.6794)
  point P24 (11.8719, -72.8214)
  point P25 (19.7424, -82.5579)
  point P26 (23.6306, -79.4143)
  point P27 (27.9992, -37.862)
  point P28 (35.9156, -36.6156)
  point P29 (35.1371, -31.6766)
  point P30 (27.2212, -32.9255)
  dimension "d50" = 5
  dimension "d51" = 5
  dimension "d52" = 5
  dimension "d53" = 5
  dimension "d54" = 5
  dimension "d55" = 5
  constraints: 54 end point, 43 point on circle, 24 tangent, 12 centre point, 6 midpoint, 6 parallel
  measures "d50" diameter of A53
  measures "d51" diameter of A57
  measures "d52" diameter of A59
  measures "d53" diameter of A62
  measures "d54" diameter of A66
  measures "d55" diameter of A69
extrude "Extrusion9" add sketch "Sketch11" against normal blind 5 contours A68 L57 A0 L56 A1 | L47 A58 A3 L48 A2 | A56 L45 A4 L42 A5 | L42 A4 L44 A56 A5 | A6 A65 L54 A7 L53 | A8 A61 L51 A9 L50 | L41 A53 A11 L38 A10 | L38 A11 A53 L40 A10
sketch "Sketch12" plane through (0, 0, 5) normal (0, 0, 1) x (1, 0, 0)
  line L0 (-133.6423, 43.9922) -> (-138.6873, 49.6358) projected
  arc A0 (-138.1583, 54.1018) -> (-138.6873, 49.6358) centre (-136.4507, 51.6352) ccw projected
  arc A1 (-131.6901, 57.863) -> (-138.1583, 54.1018) centre (-111.1209, 15.0476) ccw projected
  arc A2 (-127.6054, 56.2727) -> (-131.6901, 57.863) centre (-130.391, 55.1589) ccw projected
  line L1 (-127.6054, 56.2727) -> (-124.8131, 49.2897) projected
  arc A3 (-126.2627, 45.4898) -> (-124.8131, 49.2897) centre (-127.5987, 48.1759) ccw projected
  arc A4 (-126.2627, 45.4898) -> (-129.7609, 43.4826) centre (-111.1209, 15.0476) ccw projected
  arc A5 (-133.6423, 43.9922) -> (-129.7609, 43.4826) centre (-131.4057, 45.9916) ccw projected
  line L2 (-106.0258, -27.2686) -> (-104.3332, -25.9226) projected
  arc A6 (-101.209, -26.8039) -> (-104.3332, -25.9226) centre (-103.0884, -27.488) ccw projected
  line L3 (-101.209, -26.8039) -> (-100.5109, -28.722) projected
  arc A7 (-102.8557, -31.3511) -> (-100.5109, -28.722) centre (-102.3903, -29.406) ccw projected
  line L4 (-102.8557, -31.3511) -> (-105.2464, -30.7791) projected
  arc A8 (-106.0258, -27.2686) -> (-105.2464, -30.7791) centre (-104.781, -28.834) ccw projected
  line L5 (-157.4387, 27.5293) -> (-156.8288, 30.9169) projected
  arc A9 (-153.9152, 32.325) -> (-156.8288, 30.9169) centre (-154.8605, 30.5625) ccw projected
  line L6 (-153.9152, 32.325) -> (-151.8879, 31.2378) projected
  arc A10 (-151.5185, 27.9681) -> (-151.8879, 31.2378) centre (-152.8332, 29.4752) ccw projected
  line L7 (-151.5185, 27.9681) -> (-154.1556, 25.6678) projected
  arc A11 (-157.4387, 27.5293) -> (-154.1556, 25.6678) centre (-155.4703, 27.175) ccw projected
  arc A12 (-90.0456, 57.6162) -> (-96.9917, 60.3976) centre (-111.1209, 15.0476) ccw projected
  arc A13 (-88.7839, 53.4184) -> (-90.0456, 57.6162) centre (-91.3766, 54.9277) ccw projected
  line L8 (-88.7839, 53.4184) -> (-92.5675, 46.9188) projected
  arc A14 (-96.4543, 45.7216) -> (-92.5675, 46.9188) centre (-95.1602, 48.4281) ccw projected
  arc A15 (-96.4543, 45.7216) -> (-100.1898, 47.2425) centre (-111.1209, 15.0476) ccw projected
  arc A16 (-102.1778, 50.6148) -> (-100.1898, 47.2425) centre (-99.2253, 50.0833) ccw projected
  line L9 (-102.1778, 50.6148) -> (-100.8366, 58.0649) projected
  arc A17 (-96.9917, 60.3976) -> (-100.8366, 58.0649) centre (-97.8841, 57.5334) ccw projected
  line L10 (-95.9356, -26.6736) -> (-98.5078, -19.6065) projected
  arc A18 (-96.9399, -15.8539) -> (-98.5078, -19.6065) centre (-95.6887, -18.5805) ccw projected
  arc A19 (-96.9399, -15.8539) -> (-89.1077, -10.8642) centre (-111.1209, 15.0476) ccw projected
  arc A20 (-85.044, -11.0292) -> (-89.1077, -10.8642) centre (-87.1654, -13.1505) ccw projected
  line L11 (-85.044, -11.0292) -> (-79.7262, -16.347) projected
  arc A21 (-79.874, -20.7279) -> (-79.7262, -16.347) centre (-81.8475, -18.4683) ccw projected
  arc A22 (-91.9027, -28.391) -> (-79.874, -20.7279) centre (-111.1209, 15.0476) ccw projected
  arc A23 (-95.9356, -26.6736) -> (-91.9027, -28.391) centre (-93.1165, -25.6475) ccw projected
  line L12 (-142.415, 46.3035) -> (-137.3699, 40.6598) projected
  arc A24 (-137.2969, 36.7459) -> (-137.3699, 40.6598) centre (-139.6066, 38.6604) ccw projected
  arc A25 (-137.2969, 36.7459) -> (-139.6821, 33.4936) centre (-111.1209, 15.0476) ccw projected
  arc A26 (-143.6201, 32.4774) -> (-139.6821, 33.4936) centre (-142.2023, 35.1212) ccw projected
  line L13 (-143.6201, 32.4774) -> (-150.2477, 36.0318) projected
  arc A27 (-151.372, 40.2685) -> (-150.2477, 36.0318) centre (-148.8299, 38.6756) ccw projected
  arc A28 (-146.9121, 46.2764) -> (-151.372, 40.2685) centre (-111.1209, 15.0476) ccw projected
  arc A29 (-142.415, 46.3035) -> (-146.9121, 46.2764) centre (-144.6516, 44.3041) ccw projected
  line L14 (-73.8849, -9.1337) -> (-80.1922, -5.0377) projected
  arc A30 (-81.1985, -1.0971) -> (-80.1922, -5.0377) centre (-78.5583, -2.5216) ccw projected
  arc A31 (-81.1985, -1.0971) -> (-79.101, 3.6139) centre (-111.1209, 15.0476) ccw projected
  arc A32 (-75.4993, 5.5029) -> (-79.101, 3.6139) centre (-76.2757, 2.6051) ccw projected
  line L15 (-75.4993, 5.5029) -> (-68.2349, 3.5564) projected
  arc A33 (-66.1726, -0.3114) -> (-68.2349, 3.5564) centre (-69.0114, 0.6586) ccw projected
  arc A34 (-69.6306, -8.0782) -> (-66.1726, -0.3114) centre (-111.1209, 15.0476) ccw projected
  arc A35 (-73.8849, -9.1337) -> (-69.6306, -8.0782) centre (-72.251, -6.6176) ccw projected
  line L16 (-105.7575, 58.9508) -> (-107.0987, 51.5007) projected
  arc A36 (-110.138, 49.0334) -> (-107.0987, 51.5007) centre (-110.0513, 52.0322) ccw projected
  arc A37 (-110.138, 49.0334) -> (-114.1693, 48.9107) centre (-111.1209, 15.0476) ccw projected
  arc A38 (-117.3946, 51.3883) -> (-114.1693, 48.9107) centre (-114.4383, 51.8986) ccw projected
  line L17 (-117.3946, 51.3883) -> (-118.674, 58.7992) projected
  arc A39 (-116.0276, 62.2935) -> (-118.674, 58.7992) centre (-115.7177, 59.3096) ccw projected
  arc A40 (-108.5476, 62.4779) -> (-116.0276, 62.2935) centre (-111.1209, 15.0476) ccw projected
  arc A41 (-105.7575, 58.9508) -> (-108.5476, 62.4779) centre (-108.7101, 59.4823) ccw projected
  line L18 (-109.2411, -23.4372) -> (-116.4198, -29.1459) projected
  line L19 (-116.4198, -29.1459) -> (-110.7406, -35.6566) projected
  line L20 (-110.7406, -35.6566) -> (-109.3514, -43.5351) projected
  line L21 (-109.3514, -43.5351) -> (-97.11, -41.3766) projected
  line L22 (-97.11, -41.3766) -> (-97.5133, -39.0895) projected
  arc A42 (-96.1, -36.8212) -> (-97.5133, -39.0895) centre (-95.5437, -38.7422) ccw projected
  arc A43 (-96.1, -36.8212) -> (-86.4521, -32.9883) centre (-111.1209, 15.0476) ccw projected
  arc A44 (-83.8674, -33.6684) -> (-86.4521, -32.9883) centre (-85.5384, -34.7674) ccw projected
  line L23 (-83.8674, -33.6684) -> (-82.5913, -35.6087) projected
  line L24 (-82.5913, -35.6087) -> (-75.9074, -31.2126) projected
  line L25 (-75.9074, -31.2126) -> (-77.1835, -29.2723) projected
  arc A45 (-76.7843, -26.6297) -> (-77.1835, -29.2723) centre (-75.5126, -28.1733) ccw projected
  arc A46 (-76.7843, -26.6297) -> (-69.4435, -19.2889) centre (-111.1209, 15.0476) ccw projected
  arc A47 (-66.8009, -18.8897) -> (-69.4435, -19.2889) centre (-67.8999, -20.5607) ccw projected
  line L26 (-66.8009, -18.8897) -> (-64.8606, -20.1658) projected
  line L27 (-64.8606, -20.1658) -> (-60.4645, -13.4819) projected
  line L28 (-60.4645, -13.4819) -> (-62.4048, -12.2058) projected
  arc A48 (-63.0849, -9.6211) -> (-62.4048, -12.2058) centre (-61.3058, -10.5348) ccw projected
  arc A49 (-63.0849, -9.6211) -> (-59.252, 0.0268) centre (-111.1209, 15.0476) ccw projected
  arc A50 (-56.9837, 1.4401) -> (-59.252, 0.0268) centre (-57.331, -0.5295) ccw projected
  line L29 (-56.9837, 1.4401) -> (-54.6966, 1.0368) projected
  line L30 (-54.6966, 1.0368) -> (-53.1836, 9.6177) projected
  line L31 (-53.1836, 9.6177) -> (-61.2813, 11.0455) projected
  line L32 (-61.2813, 11.0455) -> (-77.155, 49.6681) projected
  line L33 (-77.155, 49.6681) -> (-73.3032, 53.5941) projected
  line L34 (-73.3032, 53.5941) -> (-70.7568, 56.6069) projected
  line L35 (-70.7568, 56.6069) -> (-76.8667, 61.7711) projected
  line L36 (-76.8667, 61.7711) -> (-77.6593, 60.8333) projected
  arc A51 (-81.5911, 60.2582) -> (-77.6593, 60.8333) centre (-79.9505, 62.7699) ccw projected
  arc A52 (-81.5911, 60.2582) -> (-91.9272, 65.5214) centre (-111.1209, 15.0476) ccw projected
  arc A53 (-93.4239, 66.7663) -> (-91.9272, 65.5214) centre (-90.8609, 68.3255) ccw projected
  line L37 (-93.4239, 66.7663) -> (-109.6704, 69.691) projected
  arc A54 (-111.5072, 69.0463) -> (-109.6704, 69.691) centre (-111.5287, 72.0462) ccw projected
  arc A55 (-111.5072, 69.0463) -> (-123.03, 67.7181) centre (-111.1209, 15.0476) ccw projected
  arc A56 (-126.5143, 69.6282) -> (-123.03, 67.7181) centre (-123.6916, 70.6442) ccw projected
  line L38 (-126.5143, 69.6282) -> (-126.9302, 70.7836) projected
  line L39 (-126.9302, 70.7836) -> (-134.4575, 68.0744) projected
  line L40 (-134.4575, 68.0744) -> (-134.0416, 66.919) projected
  arc A57 (-135.5094, 63.2264) -> (-134.0416, 66.919) centre (-136.8643, 65.903) ccw projected
  arc A58 (-135.5094, 63.2264) -> (-145.2356, 56.9067) centre (-111.1209, 15.0476) ccw projected
  arc A59 (-147.062, 56.233) -> (-145.2356, 56.9067) centre (-147.1309, 59.2322) ccw projected
  line L41 (-147.062, 56.233) -> (-157.7182, 43.6255) projected
  arc A60 (-158.0782, 41.7123) -> (-157.7182, 43.6255) centre (-160.687, 43.1937) ccw projected
  arc A61 (-158.0782, 41.7123) -> (-162.6893, 31.0692) centre (-111.1209, 15.0476) ccw projected
  arc A62 (-166.0858, 29.0068) -> (-162.6893, 31.0692) centre (-165.5542, 31.9593) ccw projected
  line L42 (-166.0858, 29.0068) -> (-167.2943, 29.2243) projected
  line L43 (-167.2943, 29.2243) -> (-168.7116, 21.3509) projected
  line L44 (-168.7116, 21.3509) -> (-164.8292, 20.652) projected
  line L45 (-164.8292, 20.652) -> (-159.3589, 20.0812) projected
  line L46 (-159.3589, 20.0812) -> (-156.5913, 16.9083) projected
  line L47 (-156.5913, 16.9083) -> (-148.6326, 23.8505) projected
  arc A63 (-142.0197, 20.4732) -> (-148.6326, 23.8505) centre (-146.0032, 20.8361) ccw projected
  line L48 (-142.0197, 20.4732) -> (-143.6917, 2.1197) projected
  line L49 (-143.6917, 2.1197) -> (-129.0063, -14.7161) projected
  line L50 (-129.0063, -14.7161) -> (-111.3679, -16.323) projected
  arc A64 (-109.2411, -23.4372) -> (-111.3679, -16.323) centre (-111.7308, -20.3065) ccw projected
  line L51 (-130.2826, 31.873) -> (-125.239, 23.425) projected
  arc A65 (-126.0322, 21.9145) -> (-125.239, 23.425) centre (-126.0977, 22.9124) ccw projected
  line L52 (-126.0322, 21.9145) -> (-135.8502, 21.2706) projected
  arc A66 (-137.3807, 23.2128) -> (-135.8502, 21.2706) centre (-135.9484, 22.7674) ccw projected
  arc A67 (-132.7503, 32.0305) -> (-137.3807, 23.2128) centre (-111.1209, 15.0476) ccw projected
  arc A68 (-130.2826, 31.873) -> (-132.7503, 32.0305) centre (-131.5705, 31.1041) ccw projected
  line L53 (-136.5676, 13.3956) -> (-127.0276, 10.9882) projected
  arc A69 (-126.5204, 9.3593) -> (-127.0276, 10.9882) centre (-127.2722, 10.0186) ccw projected
  line L54 (-126.5204, 9.3593) -> (-133.0075, 1.9617) projected
  arc A70 (-135.463, 2.2527) -> (-133.0075, 1.9617) centre (-134.1353, 2.9506) ccw projected
  arc A71 (-138.4239, 11.762) -> (-135.463, 2.2527) centre (-111.1209, 15.0476) ccw projected
  arc A72 (-136.5676, 13.3956) -> (-138.4239, 11.762) centre (-136.9346, 11.9412) ccw projected
  line L55 (-127.9462, -4.1141) -> (-119.4982, 0.9295) projected
  arc A73 (-117.9877, 0.1363) -> (-119.4982, 0.9295) centre (-118.9856, 0.0708) ccw projected
  line L56 (-117.9877, 0.1363) -> (-117.3438, -9.6817) projected
  arc A74 (-119.286, -11.2122) -> (-117.3438, -9.6817) centre (-118.8406, -9.7799) ccw projected
  arc A75 (-128.1037, -6.5818) -> (-119.286, -11.2122) centre (-111.1209, 15.0476) ccw projected
  arc A76 (-127.9462, -4.1141) -> (-128.1037, -6.5818) centre (-127.1773, -5.402) ccw projected
  line L57 (-109.4688, -10.3991) -> (-107.0615, -0.8591) projected
  arc A77 (-105.4325, -0.3519) -> (-107.0615, -0.8591) centre (-106.0918, -1.1038) ccw projected
  line L58 (-105.4325, -0.3519) -> (-98.0349, -6.839) projected
  arc A78 (-98.326, -9.2945) -> (-98.0349, -6.839) centre (-99.0239, -7.9668) ccw projected
  arc A79 (-107.8352, -12.2554) -> (-98.326, -9.2945) centre (-111.1209, 15.0476) ccw projected
  arc A80 (-109.4688, -10.3991) -> (-107.8352, -12.2554) centre (-108.0144, -10.7661) ccw projected
  line L59 (-91.9591, -1.7778) -> (-97.0027, 6.6703) projected
  arc A81 (-96.2095, 8.1808) -> (-97.0027, 6.6703) centre (-96.1441, 7.1829) ccw projected
  line L60 (-96.2095, 8.1808) -> (-86.3915, 8.8246) projected
  arc A82 (-84.861, 6.8825) -> (-86.3915, 8.8246) centre (-86.2933, 7.3279) ccw projected
  arc A83 (-89.4914, -1.9352) -> (-84.861, 6.8825) centre (-111.1209, 15.0476) ccw projected
  arc A84 (-91.9591, -1.7778) -> (-89.4914, -1.9352) centre (-90.6712, -1.0088) ccw projected
  line L61 (-85.6741, 16.6997) -> (-95.2141, 19.107) projected
  arc A85 (-95.7213, 20.736) -> (-95.2141, 19.107) centre (-94.9695, 20.0766) ccw projected
  line L62 (-95.7213, 20.736) -> (-89.2342, 28.1336) projected
  arc A86 (-86.7787, 27.8425) -> (-89.2342, 28.1336) centre (-88.1064, 27.1446) ccw projected
  arc A87 (-83.8178, 18.3333) -> (-86.7787, 27.8425) centre (-111.1209, 15.0476) ccw projected
  arc A88 (-85.6741, 16.6997) -> (-83.8178, 18.3333) centre (-85.3071, 18.1541) ccw projected
  line L63 (-94.2955, 34.2094) -> (-102.7435, 29.1658) projected
  arc A89 (-104.254, 29.959) -> (-102.7435, 29.1658) centre (-103.2561, 30.0244) ccw projected
  line L64 (-104.254, 29.959) -> (-104.8979, 39.777) projected
  arc A90 (-102.9557, 41.3075) -> (-104.8979, 39.777) centre (-103.4011, 39.8751) ccw projected
  arc A91 (-94.138, 36.6771) -> (-102.9557, 41.3075) centre (-111.1209, 15.0476) ccw projected
  arc A92 (-94.2955, 34.2094) -> (-94.138, 36.6771) centre (-95.0644, 35.4973) ccw projected
  line L65 (-112.7729, 40.4944) -> (-115.1802, 30.9544) projected
  arc A93 (-116.8092, 30.4472) -> (-115.1802, 30.9544) centre (-116.1499, 31.199) ccw projected
  line L66 (-116.8092, 30.4472) -> (-124.2068, 36.9342) projected
  arc A94 (-123.9157, 39.3898) -> (-124.2068, 36.9342) centre (-123.2178, 38.062) ccw projected
  arc A95 (-114.4065, 42.3506) -> (-123.9157, 39.3898) centre (-111.1209, 15.0476) ccw projected
  arc A96 (-112.7729, 40.4944) -> (-114.4065, 42.3506) centre (-114.2273, 40.8614) ccw projected
  circle A97 centre (-100.8802, 2.7542) radius 2 projected
  circle A98 centre (-121.3615, 27.3411) radius 2 projected
  circle A99 centre (-126.059, 16.4085) radius 1.5 projected
  circle A100 centre (-96.1827, 13.6868) radius 1.5 projected
  circle A101 centre (-112.4817, 0.1095) radius 1.5 projected
  circle A102 centre (-109.76, 29.9858) radius 1.5 projected
  circle A103 centre (-123.4143, 4.807) radius 2 projected
  circle A104 centre (-98.8274, 25.2883) radius 2 projected
  circle A105 centre (-111.1209, 15.0476) radius 12 projected
  circle A106 centre (-129.3392, 65.6653) radius 1.55 projected
  circle A107 centre (-57.4488, 5.5838) radius 1.55 projected
  circle A108 centre (-81.1726, -30.4864) radius 1.55 projected
  circle A109 centre (-101.657, -38.6244) radius 1.55 projected
  circle A110 centre (-65.5868, -14.9006) radius 1.55 projected
  circle A111 centre (-76.3938, 56.134) radius 1.55 projected
  circle A112 centre (-164.0662, 24.5789) radius 1.55 projected
  arc A113 (-21.8035, -78.1288) -> (-9.3616, -79.8626) centre (-10.3402, -41.375) ccw projected
  line L67 (-9.3616, -79.8626) -> (-9.1582, -87.86) projected
  arc A114 (-24.6798, -85.6088) -> (-9.1582, -87.86) centre (-10.3402, -41.375) ccw projected
  line L68 (-24.6798, -85.6088) -> (-21.8314, -78.2051) projected
  arc A115 (-21.8314, -78.2051) -> (-21.8035, -78.1288) centre (-24.1646, -77.3074) ccw projected
  arc A116 (1.123, -4.6212) -> (-11.3188, -2.8874) centre (-10.3402, -41.375) ccw projected
  line L69 (-11.3188, -2.8874) -> (-11.6366, 9.6085) projected
  arc A117 (5.6174, 7.0642) -> (-11.6366, 9.6085) centre (-10.3402, -41.375) ccw projected
  line L70 (5.6174, 7.0642) -> (1.1509, -4.5449) projected
  arc A118 (1.1509, -4.5449) -> (1.123, -4.6212) centre (3.4842, -5.4426) ccw projected
  arc A119 (4.1075, -90.2858) -> (19.7424, -82.5579) centre (-10.3402, -41.375) ccw projected
  line L71 (4.1075, -90.2858) -> (0.5664, -78.2978) projected
  arc A120 (0.5664, -78.2978) -> (11.8719, -72.8214) centre (-10.3402, -41.375) ccw projected
  arc A121 (11.8719, -72.8214) -> (11.9219, -72.8853) centre (13.8659, -71.3135) ccw projected
  line L72 (11.9219, -72.8853) -> (19.7424, -82.5579) projected
  arc A122 (-59.922, -29.4317) -> (-61.047, -46.8359) centre (-10.3402, -41.375) ccw projected
  line L73 (-59.922, -29.4317) -> (-47.7696, -32.359) projected
  arc A123 (-47.7696, -32.359) -> (-48.6796, -44.888) centre (-10.3402, -41.375) ccw projected
  arc A124 (-48.6796, -44.888) -> (-48.76, -44.8994) centre (-48.3708, -47.3689) ccw projected
  line L74 (-48.76, -44.8994) -> (-61.047, -46.8359) projected
  arc A125 (-36.4384, -13.0706) -> (-44.1607, -22.9787) centre (-10.3402, -41.375) ccw projected
  line L75 (-44.1607, -22.9787) -> (-55.1414, -17.0059) projected
  arc A126 (-44.311, -3.3357) -> (-55.1414, -17.0059) centre (-10.3402, -41.375) ccw projected
  line L76 (-44.311, -3.3357) -> (-36.4904, -13.0083) projected
  arc A127 (-36.4904, -13.0083) -> (-36.4384, -13.0706) centre (-34.5464, -11.4365) ccw projected
  arc A128 (34.8667, -52.2645) -> (35.9156, -36.6156) centre (-10.3402, -41.375) ccw projected
  line L77 (34.8667, -52.2645) -> (27.0892, -50.391) projected
  arc A129 (27.0892, -50.391) -> (27.9992, -37.862) centre (-10.3402, -41.375) ccw projected
  arc A130 (27.9992, -37.862) -> (28.0796, -37.8506) centre (27.6903, -35.3811) ccw projected
  line L78 (28.0796, -37.8506) -> (35.9156, -36.6156) projected
  arc A131 (-26.4675, -76.3344) -> (-26.4979, -76.4097) centre (-24.1646, -77.3074) ccw projected
  line L79 (-26.4979, -76.4097) -> (-29.3464, -83.8134) projected
  arc A132 (-42.3743, -75.0806) -> (-29.3464, -83.8134) centre (-10.3402, -41.375) ccw projected
  line L80 (-42.3743, -75.0806) -> (-36.863, -69.2818) projected
  arc A133 (-36.863, -69.2818) -> (-26.4675, -76.3344) centre (-10.3402, -41.375) ccw projected
  arc A134 (5.7871, -6.4156) -> (5.8175, -6.3403) centre (3.4842, -5.4426) ccw projected
  line L81 (5.8175, -6.3403) -> (10.2839, 5.2688) projected
  arc A135 (24.7939, -4.4075) -> (10.2839, 5.2688) centre (-10.3402, -41.375) ccw projected
  line L82 (24.7939, -4.4075) -> (16.1826, -13.4682) projected
  arc A136 (16.1826, -13.4682) -> (5.7871, -6.4156) centre (-10.3402, -41.375) ccw projected
  line L83 (23.6306, -79.4143) -> (15.81, -69.7417) projected
  arc A137 (15.81, -69.7417) -> (15.7579, -69.6794) centre (13.8659, -71.3135) ccw projected
  arc A138 (15.7579, -69.6794) -> (23.4803, -59.7713) centre (-10.3402, -41.375) ccw projected
  line L84 (23.4803, -59.7713) -> (34.461, -65.7441) projected
  arc A139 (23.6306, -79.4143) -> (34.461, -65.7441) centre (-10.3402, -41.375) ccw projected
  line L85 (-60.2686, -51.7749) -> (-47.9816, -49.8384) projected
  arc A140 (-47.9816, -49.8384) -> (-47.9016, -49.8245) centre (-48.3708, -47.3689) ccw projected
  arc A141 (-47.9016, -49.8245) -> (-43.1821, -61.4663) centre (-10.3402, -41.375) ccw projected
  line L86 (-43.1821, -61.4663) -> (-53.8451, -67.9894) projected
  arc A142 (-60.2686, -51.7749) -> (-53.8451, -67.9894) centre (-10.3402, -41.375) ccw projected
  arc A143 (-32.5523, -9.9286) -> (-32.6023, -9.8647) centre (-34.5464, -11.4365) ccw projected
  line L87 (-32.6023, -9.8647) -> (-40.4229, -0.1921) projected
  arc A144 (-24.7879, 7.5358) -> (-40.4229, -0.1921) centre (-10.3402, -41.375) ccw projected
  line L88 (-24.7879, 7.5358) -> (-21.2468, -4.4522) projected
  arc A145 (-21.2468, -4.4522) -> (-32.5523, -9.9286) centre (-10.3402, -41.375) ccw projected
  line L89 (35.1371, -31.6766) -> (27.3011, -32.9116) projected
  arc A146 (27.3011, -32.9116) -> (27.2212, -32.9255) centre (27.6903, -35.3811) ccw projected
  arc A147 (27.2212, -32.9255) -> (22.5017, -21.2837) centre (-10.3402, -41.375) ccw projected
  line L90 (22.5017, -21.2837) -> (29.326, -17.1089) projected
  arc A148 (35.1371, -31.6766) -> (29.326, -17.1089) centre (-10.3402, -41.375) ccw projected
  circle A149 centre (-81.1726, -30.4864) radius 2.1 projected
  circle A150 centre (-65.5868, -14.9006) radius 2.1 projected
  circle A151 centre (-101.657, -38.6244) radius 2.1 projected
  circle A152 centre (-57.4488, 5.5838) radius 2.1 projected